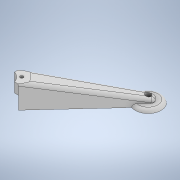
# Autodesk Inventor part: Noga
Saved by Autodesk Inventor 2020 (Build 240168000, 168)
## iProperties
Created: 2021-03-05
Part Number: Noga
Material: Generic
Document SubType Name: Modeling
Designer: patry
Density: 1 g/cm^3
Appearance: Default
Author: patry
Autodesk Inventor part; units mm, degrees
ref_plane "YZ Plane" through (0, 0, 0) normal (1, 0, 0) x (0, 1, 0)
ref_plane "XZ Plane" through (0, 0, 0) normal (0, 1, 0) x (-1, 0, 0)
ref_plane "XY Plane" through (0, 0, 0) normal (0, 0, 1) x (1, 0, 0)
sketch "Sketch1" plane through (0, 0, 0) normal (0, 1, 0) x (-1, 0, 0)
  arc A0 (5, 25) -> (25, 5) centre (25, 25) ccw
  circle A1 centre (25, 25) radius 20
  arc A2 (0, 10) -> (10, 0) centre (10, 10) ccw
  circle A3 centre (10, 10) radius 10
  line L0 (5.8856, 19.1144) -> (0, 19.1144)
  line L1 (0, 90) -> (0, 10)
  line L2 (19.1144, 5.8856) -> (19.1144, 0)
  line L3 (10, 0) -> (190, 0)
  line L4 (0, 19.1144) -> (19.1144, 19.1144)
  line L5 (19.1144, 19.1144) -> (19.1144, 0)
  line L6 (19.1144, 0) -> (0, 0)
  line L7 (0, 0) -> (0, 19.1144)
  arc A4 (45, 75) -> (5, 75) centre (25, 75) ccw
  circle A5 centre (25, 75) radius 20
  line L8 (25, 75) -> (25, 25)
  line L9 (25, 75) -> (35, 75)
  line L10 (35, 75) -> (35, 50)
  line L11 (35, 50) -> (25, 50)
  line L12 (25, 50) -> (25, 75)
  circle A6 centre (25, 75) radius 20
  line L13 (19.1144, 80.8856) -> (19.1144, 100)
  line L14 (0, 80.8856) -> (19.1144, 80.8856)
  line L15 (0, 100) -> (0, 80.8856)
  line L16 (19.1144, 100) -> (0, 100)
  circle A7 centre (10, 90) radius 10
  line L17 (19.1144, 0) -> (169.1144, 0) construction
  line L18 (-101.8121, -91.2055) -> (-91.2055, -101.8121)
  line L19 (0, 0) -> (-96.5088, -96.5088)
  line L20 (-96.5088, -96.5088) -> (-91.2055, -101.8121)
  line L21 (-91.2055, -101.8121) -> (-101.8121, -91.2055)
  line L22 (-91.2055, -101.8121) -> (10.6066, 0)
  line L23 (-101.8121, -91.2055) -> (0, 10.6066)
  line L24 (0, 19.1144) -> (-101.8121, -91.2055)
  line L25 (19.1144, 0) -> (-91.2055, -101.8121)
  point P0 (19.1144, 5.8856)
  point P1 (5.8856, 19.1144)
  point P2 (10, 100)
  point P3 (5.8856, 80.8856)
  point P4 (19.1144, 94.1144)
  point P5 (5.8856, 19.1144)
  point P6 (19.1144, 5.8856)
  dimension "d0" = 10
  dimension "d1" = 25
  constraints: 52 end point, 10 point on circle, 8 centre point, 6 symmetric about line, 4 horizontal, 4 parallel, 4 point on line, 3 coincident, 3 perpendicular, 1 midpoint, 1 vertical, 2 other
  measures "d0" distance of L10.end L11.end
  measures "d1" distance of L9.end L10.end
extrude "Extrusion1" add sketch "Sketch1" along normal blind 35 contours A0 A3 A2 | A3 L1 L0 | L2 L3 A3 | L7 L19 L18 L23 L1 | A2 L6 L7 | L1 L23 L24 | L3 L22 L18 L19 L6 | L25 L22 L3
sketch "Sketch3" plane through (0, 0, 0) normal (0, -1, 0) x (1, 0, 0)
  arc A0 (-19.1144, 5.8856) -> (-5.8856, 19.1144) centre (-25, 25) ccw projected
  circle A1 centre (-25, 25) radius 20
  line L0 (0, 0) -> (-19.1144, 0)
  line L1 (-19.1144, 0) -> (-19.1144, 19.1144)
  line L2 (-19.1144, 19.1144) -> (0, 19.1144)
  line L3 (0, 19.1144) -> (0, 0)
  line L4 (91.2055, -101.8121) -> (-19.1144, 0) projected
  line L5 (-5.8856, 19.1144) -> (0, 19.1144) projected
  line L6 (-19.1144, 0) -> (0, 19.1144)
  line L7 (-19.1144, 19.1144) -> (0, 0)
  point P0 (-5.8856, 19.1144)
  point P1 (-19.1144, 5.8856)
  constraints: 12 end point, 2 parallel, 1 centre point, 1 coincident, 1 horizontal, 1 perpendicular
extrude "Extrusion4" cut sketch "Sketch3" against normal blind 20 contours A0 L7 L6 L1 | A0 L2 L6 L7 | L6 L7 L0 | L6 L3 L7
fillet "Fillet2" radius 10 1 edges at (0, 10, 0)
sketch "Sketch6" plane through (91.2055, 0, -101.8121) normal (-0.6782, 0, -0.7349) x (-0.7349, 0, 0.6782)
  line L0 (150.1206, 20) -> (150.1206, 35) projected
  line L1 (150.1206, 35) -> (136.6046, 35)
  line L2 (0, 35) -> (150.1206, 35) projected
  line L3 (143.4227, 0) -> (150.1206, 0) projected
  line L4 (0, 35) -> (150.1206, 35)
  line L5 (150.1206, 35) -> (150.1206, 0)
  line L6 (150.1206, 0) -> (0, 0)
  line L7 (0, 0) -> (0, 35)
  line L8 (0, 0) -> (150.1206, 0) projected
  line L9 (0, 0) -> (0, 10)
  line L10 (0, 0) -> (10, 0) construction
  line L11 (0, 10) -> (136.6046, 35)
  line L12 (0, 10) -> (-15.7766, 7.1127)
  line L13 (-15.7766, 7.1127) -> (-15.4206, 35)
  line L14 (0, 0) -> (0, 35) projected
  line L15 (-15.4206, 35) -> (0, 35)
  point P0 (136.0739, 0)
  dimension "d22" = 13.516
  dimension "d23" = 10
  dimension "d24" = 90
  constraints: 22 end point, 3 perpendicular, 2 horizontal, 2 parallel, 1 point on line, 1 vertical
  measures "d22" distance of L0.end L1.end
  measures "d23" distance of L6.end L9.end
  measures "d24" angle of L10 L9
extrude "Extrusion5" cut sketch "Sketch6" against normal through all contours L11 L7 L2 | L7 L12 L13 L15
sketch "Sketch7" plane through (0, 20, 0) normal (0, -1, 0) x (1, 0, 0)
  line L0 (0, 0) -> (200, 0)
  line L1 (200, 0) -> (200, 100)
  line L2 (200, 100) -> (0, 100)
  line L3 (0, 100) -> (0, 0)
  line L4 (0, 0) -> (7, 0)
  line L5 (7, 0) -> (7, 7)
  line L6 (7, 7) -> (0, 7)
  line L7 (0, 7) -> (0, 0)
  line L8 (200, 100) -> (193, 100)
  line L9 (193, 100) -> (193, 93)
  line L10 (193, 93) -> (200, 93)
  line L11 (200, 93) -> (200, 100)
  line L12 (7, 7) -> (193, 7)
  line L13 (193, 7) -> (193, 93)
  line L14 (193, 93) -> (7, 93)
  line L15 (7, 93) -> (7, 7)
  line L16 (0, 0) -> (-200, 0)
  line L17 (-200, 0) -> (-200, 100)
  line L18 (-200, 100) -> (0, 100)
  line L19 (0, 0) -> (-7, 0)
  line L20 (-7, 0) -> (-7, 7)
  line L21 (-7, 7) -> (0, 7)
  line L22 (-200, 100) -> (-193, 100)
  line L23 (-193, 100) -> (-193, 93)
  line L24 (-193, 93) -> (-200, 93)
  line L25 (-200, 93) -> (-200, 100)
  line L26 (-7, 7) -> (-193, 7)
  line L27 (-193, 7) -> (-193, 93)
  line L28 (-193, 93) -> (-7, 93)
  line L29 (-7, 93) -> (-7, 7)
  dimension "d27" = 200
  dimension "d28" = 100
  dimension "d29" = 7
  dimension "d30" = 7
  dimension "d31" = 7
  dimension "d32" = 7
  constraints: 60 end point, 9 symmetric about line, 8 parallel, 4 horizontal, 4 perpendicular
  measures "d27" distance of L2.end L1.end
  measures "d28" distance of L1.end L0.end
  measures "d29" distance of L6.end L5.end
  measures "d30" distance of L5.end L4.end
  measures "d31" distance of L10.end L9.end
  measures "d32" distance of L9.end L8.end
hole "Hole1" at (-7, 20, 7) direction (0, 1, 0) diameter 5 end through all
fillet "Fillet3" radius 5 1 edges at (96.5088, 9.945, -96.5088)
fillet "Fillet4" radius 5 4 edges at (90.3527, 9.0335, -101.025) (91.2055, 2.9156, -101.8121) (101.025, 8.9228, -90.3527) (101.8121, 2.8606, -91.2055)
sketch "Sketch8" plane through (0, 0, 0) normal (0, -1, 0) x (1, 0, 0)
  line L0 (98.4155, -94.6021) -> (94.6021, -98.4155) projected
  line L1 (98.4155, -94.6021) -> (103.9755, -89.0422)
  line L2 (0, 19.1144) -> (98.5544, -87.6756) projected
  line L3 (98.5544, -87.6756) -> (108.5515, -97.6726)
  ellipse E0 centre (94.88, -91.0666) end of major axis (91.3445, -87.531) minor radius 0.0367 (98.4155, -94.6021) -> (95.5415, -91.677) ccw projected
  line L4 (98.4155, -94.6021) -> (90.1473, -102.8703)
  line L5 (87.6756, -98.5544) -> (-19.1144, 0) projected
  line L6 (87.6756, -98.5544) -> (92.1576, -103.0365)
  circle A0 centre (90.9886, -90.9886) radius 7.8068
  circle A1 centre (90.9886, -90.9886) radius 20
  point P0 (0, 0)
  point P1 (98.0828, -94.2471)
  point P2 (96.5088, -96.5088)
  dimension "d42" = 40
  constraints: 8 end point, 3 tangent, 2 centre point, 1 coincident, 1 collinear, 1 point on line, 2 other
  measures "d42" diameter of A1
extrude "Extrusion6" add sketch "Sketch8" against normal blind 5 contours L1 L3 L2 A1 L5 L6 L4 L0 | E0 A0 L2 L3 L1 | L0 L4 L6 L5 A0 | A0 | L5 A1 L2 A0
fillet "Fillet5" radius 5 1 edges at (105.1307, 5, -105.1307)
sketch "Sketch9" plane through (0, 0, 0) normal (0, -1, 0) x (1, 0, 0)
  arc A0 (72.1624, -84.2376) -> (84.2376, -72.1624) centre (90.9886, -90.9886) ccw projected
  circle A1 centre (90.9886, -90.9886) radius 4.25
  point P0 (0, 0)
  dimension "d46" = 8.5
  constraints: 1 centre point, 1 coincident
  measures "d46" diameter of A1
extrude "Extrusion7" cut sketch "Sketch9" against normal through all
sketch "Sketch10" plane through (0, 0, 0) normal (0, -1, 0) x (1, 0, 0)
  circle A0 centre (90.9886, -90.9886) radius 4.25 projected
  circle A1 centre (90.9886, -90.9886) radius 4.25
  circle A2 centre (90.9886, -90.9886) radius 2.5
  point P0 (0, 0)
  dimension "d49" = 5
  constraints: 2 centre point, 2 coincident
  measures "d49" diameter of A2
extrude "Extrusion8" add sketch "Sketch10" against normal blind 5
body "Solid1"
